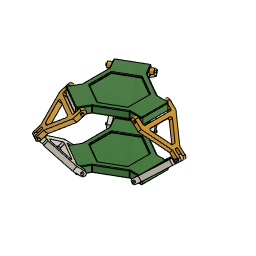
Triangular Podium v1 (Autodesk Fusion 360 design; units mm, degrees)
Autodesk Fusion 360 part; units mm, degrees
sketch "Sketch1" plane through (0, 0, 0) normal (0, 0, 1) x (1, 0, 0)
  line L0 (100, 57.735) -> (0, 115.4701)
  line L1 (0, 115.4701) -> (-100, 57.735)
  line L2 (-100, 57.735) -> (-100, -57.735)
  line L3 (-100, -57.735) -> (0, -115.4701)
  line L4 (0, -115.4701) -> (100, -57.735)
  line L5 (100, -57.735) -> (100, 57.735)
  line L6 (80, 46.188) -> (0, 92.376)
  line L7 (0, 92.376) -> (-80, 46.188)
  line L8 (-80, 46.188) -> (-80, -46.188)
  line L9 (-80, -46.188) -> (0, -92.376)
  line L10 (0, -92.376) -> (80, -46.188)
  line L11 (80, -46.188) -> (80, 46.188)
  dimension "d1" = 100
  dimension "d2" = 80
  measures "d1" distance of origin L5
  measures "d2" distance of origin L11
extrude "Extrude1" add sketch "Sketch1" along normal mid plane 20 contours L6 L7 L8 L9 L10 L11 makes body 1
extrude "Extrude2" add sketch "Sketch1" along normal mid plane 30 bodies 1
extrude "Extrude3" add 1 faces at (100, -19.245, -5) along direction (1, 0, 0) blind 50 on bodies 1 bodies 1
hole "Hole1" at (135, -57.735, 0) direction (0, 1, 0) diameter 10 end through all bodies 1
pattern_circular "C-Pattern1" count 3 over 360 about axis through (0, 0, 1.75) along (0, 0, 1) of "Extrude3", "Hole1"
fillet "Fillet1" radius 5 12 edges at (-25, -158.7713, 0) (-125, -101.0363, 0) (-100, -57.735, 0) (-100, 57.735, 0) (-125, 101.0363, 0) (-25, 158.7713, 0) (0, 115.4701, 0) (100, -57.735, 0) (0, -115.4701, 0) (150, -57.735, 0) (150, 57.735, 0) (100, 57.735, 0) on bodies 1
fillet "Fillet2" radius 2.5 2 faces at (-74.0032, -93.0206, 15) (-74.0032, -93.0206, -15) on bodies 1
cylinder "CylinderPrimitive1" add diameter 10 height -115.47 placed x (1, 0, 0) y (0, 0, 1) z (0, -1, 0) at (135, -57.735, 0) separate body makes body 2
move_face "OffsetFaces1" offset 20 1 faces at (136.3101, -57.735, -1.9935) on bodies 2
move_face "OffsetFaces2" offset 20 1 faces at (136.3101, 57.735, -1.9935) on bodies 2
pattern_circular "C-Pattern2" count 3 over 360 about axis through (0, 0, 1.75) along (0, 0, 1) of bodies 2 makes body 3 at (-45.856, 131.2484, 4.7396) makes body 4 at (-44.3828, -128.6965, 4.8131)
copy_body "Body->Comp1" bodies 1 removing the originals makes body 5 in component "Component"
copy_body "CutPasteBodies1" bodies 2 3 4 removing the originals makes body 6 makes body 7 makes body 8 in component "Component"
sketch "Sketch3" plane through (150, 0, 0) normal (1, 0, 0) x (0, 1, 0)
  line L0 (-52.735, -12.5) -> (52.735, -12.5)
  line L1 (52.735, -12.5) -> (52.735, 12.5)
  line L2 (52.735, 12.5) -> (-52.735, 12.5)
  line L3 (-52.735, 12.5) -> (-52.735, -12.5)
  line L4 (-77.735, 5) -> (-77.735, -5)
  line L5 (-57.735, 12.5) -> (-57.735, -12.5)
  line L6 (-52.735, -15) -> (52.735, -15)
  line L7 (57.735, -12.5) -> (57.735, 12.5)
  line L8 (77.735, -5) -> (77.735, 5)
  line L9 (-57.735, -15) -> (-72.735, -15)
  line L10 (-72.735, -15) -> (-72.735, 30)
  line L11 (-57.735, 20) -> (-57.735, -15)
  line L12 (-52.735, 25) -> (0, 25)
  line L13 (0, 25) -> (0, 100) construction
  line L14 (0, 130) -> (-15, 130)
  line L15 (-15, 130) -> (-72.735, 30)
  line L16 (0, 130) -> (15, 130)
  line L17 (15, 130) -> (72.735, 30)
  line L18 (72.735, -15) -> (72.735, 30)
  line L19 (57.735, -15) -> (72.735, -15)
  line L20 (57.735, 20) -> (57.735, -15)
  line L21 (52.735, 25) -> (0, 25)
  line L22 (40.9808, 40) -> (0, 40)
  line L23 (-40.9808, 40) -> (0, 40)
  line L24 (-6.3397, 115) -> (-45.3109, 47.5)
  line L25 (0, 115) -> (-6.3397, 115)
  line L26 (0, 115) -> (6.3397, 115)
  line L27 (6.3397, 115) -> (45.3109, 47.5)
  arc A0 (-45.3109, 47.5) -> (-40.9808, 40) centre (-40.9808, 45) ccw
  arc A1 (40.9808, 40) -> (45.3109, 47.5) centre (40.9808, 45) ccw
  arc A2 (-52.735, 25) -> (-57.735, 20) centre (-52.735, 20) ccw
  arc A3 (57.735, 20) -> (52.735, 25) centre (52.735, 20) ccw
  point P0 (-57.735, 25)
  dimension "d25" = 15
  dimension "d26" = 40
  dimension "d27" = 45
  dimension "d28" = 15
  dimension "d29" = 60
  dimension "d31" = 5
  constraint horizontal L9
  constraint vertical L10
  constraint vertical L11
  constraint vertical L5.end L9.start
  constraint horizontal L6.start L9.start
  constraint perpendicular L11 L12
  constraint perpendicular L0 L13
  constraint horizontal L14
  constraint vertical origin L14.start
  constraint symmetric L9.start L13 L19.start
  constraint symmetric L9.end L13 L18.start
  constraint symmetric L10.end L13 L17.end
  constraint symmetric L12.end L13 L21.end
  constraint symmetric L13 L14.start L16.start
  constraint symmetric L13 L14.end L16.end
  constraint tangent L23 A0
  constraint tangent L24 A0
  constraint tangent L22 A1
  constraint tangent L27 A1
  constraint equal A0 A1
  constraint coincident P0 L11
  constraint coincident P0 L12
  constraint tangent L11 A2
  constraint tangent L12 A2
  constraint equal A0 A2
  constraint tangent L20 A3
  constraint tangent L21 A3
  constraint equal A0 A3
  measures "d25" distance of L9.start L9.end
  measures "d26" distance of L9.start P0
  measures "d27" distance of L9.end L10.end
  measures "d28" distance of L14.start L14.end
  measures "d29" angle of L12 L15
  measures "d31" radius of A0
extrude "Extrude1'" add sketch "Sketch3" along normal blind 20 separate body contours L5 L7 L9 L10 L11 L12 L14 L15 L16 L17 L18 L19 L20 L21 A2 A3 makes body 9 in component "Component'"
hole "Hole1'" at (160, -72.735, 0) direction (0, 1, 0) diameter 10 end through all bodies 9 in component "Component'"
fillet "Fillet1'" radius 10 4 edges at (170, -65.235, -15) (150, -65.235, -15) (170, 65.235, -15) (150, 65.235, -15) on bodies 9 in component "Component'"
extrude "Extrude1''" add sketch "Sketch3" along normal blind 20 separate body contours L5 L7 L9 L10 L11 L12 L14 L15 L16 L17 L18 L19 L20 L21 A2 A3 makes body 10 in component "Component''"
hole "Hole1''" at (160, -72.735, 0) direction (0, 1, 0) diameter 10 end through all bodies 10 in component "Component''"
fillet "Fillet1''" radius 10 4 edges at (170, -65.235, -15) (150, -65.235, -15) (170, 65.235, -15) (150, 65.235, -15) on bodies 10 in component "Component''"
sketch "Sketch4" plane through (0, 0, 0) normal (0, 1, 0) x (1, 0, 0)
  line L0 (150, -130) -> (170, -130)
  line L1 (225, -130) -> (245, -130)
  line L2 (150, -130) -> (170, -130)
  line L3 (170, -130) -> (170, -160)
  line L4 (150, -160) -> (150, -130)
  line L5 (225, -130) -> (245, -130)
  line L6 (245, -130) -> (245, -160)
  line L7 (225, -160) -> (225, -130)
  circle A0 centre (160, -160) radius 5
  arc A1 (150, -160) -> (170, -160) centre (160, -160) ccw
  circle A2 centre (235, -160) radius 5
  arc A3 (225, -160) -> (245, -160) centre (235, -160) ccw
  dimension "d40" = 20
  dimension "d41" = 30
  dimension "d42" = 20
  dimension "d43" = 30
  dimension "d44" = 20
  dimension "d45" = 10
  dimension "d46" = 20
  dimension "d47" = 10
  constraint horizontal L2
  constraint vertical L3
  constraint vertical L4
  constraint coincident L0.start L2.start
  constraint horizontal L5
  constraint vertical L6
  constraint vertical L7
  constraint coincident L1.start L5.start
  constraint concentric A0 A1
  constraint concentric A2 A3
  measures "d40" distance of L0.start L0.end
  measures "d41" distance of L0.start L4.start
  measures "d42" distance of L1.start L1.end
  measures "d43" distance of L1.start L7.start
  measures "d44" diameter of A1
  measures "d45" diameter of A0
  measures "d46" diameter of A3
  measures "d47" diameter of A2
extrude "Extrude2'" add sketch "Sketch4" along normal mid plane 10 contours L0 L2 L3 L4 A1 bodies 9 in component "Component'"
extrude "Extrude2''" add sketch "Sketch4" along normal blind 10 from surface at 5 contours L1 L5 L6 L7 A3 sketch seen with x (1, 0, 0) y (0, 1, 0) z (0, 0, 1) at (-75, 0, 0) bodies 10 in component "Component''"
mirror "Mirror1" about plane through (-75, 0, 0) normal (0, 1, 0) of "Extrude2''" in component "Component''"
cylinder "CylinderPrimitive1'" add diameter 10 height 40 placed x (1, 0, 0) y (0, 0, 1) z (0, -1, 0) at (160, -5, 160) separate body makes body 11 in component "Component'''"
move_body "Move1" bodies 11 to x (1, 0, 0) y (0, 1, 0) z (0, 0, 1) at (0, 25, 0) in component "Component'''"
component_pattern "component pattern"
component "Component" placed x (1, 0, 0) y (0, 1, 0) z (0, 0, 1) at (0, 0, 0)
component "Component'" placed x (1, 0, 0) y (0, 1, 0) z (0, 0, 1) at (-25, 0, 0)
component "Component''" placed x (-1, 0, 0) y (0, 1, 0) z (0, 0, -1) at (295, 0, 320)
component "Component'''" placed x (-0.99999, 0, -0.004441) y (0, 1, 0) z (0.004441, 0, -0.99999) at (294.2879, 0, 320.7089)
component "Component'" placed x (-0.5, 0.866025, 0) y (-0.866025, -0.5, 0) z (0, 0, 1) at (12.5, -21.6506, 0)
component "Component''" placed x (0.5, -0.866025, 0) y (-0.866025, -0.5, 0) z (0, 0, -1) at (-147.5, 255.4775, 320)
component "Component'''" placed x (0.5, -0.866025, 0) y (-0.866025, -0.5, 0) z (0, 0, -1) at (-147.5, 255.4775, 320)
component "Component'" placed x (-0.5, -0.866025, 0) y (0.866025, -0.5, 0) z (0, 0, 1) at (12.5, 21.6506, 0)
component "Component''" placed x (0.5, 0.866025, 0) y (0.866025, -0.5, 0) z (0, 0, -1) at (-147.5, -255.4775, 320)
component "Component'''" placed x (0.5, 0.866025, 0) y (0.866025, -0.5, 0) z (0, 0, -1) at (-147.5, -255.4775, 320)
component "Component" placed x (1, 0, 0) y (0, 1, 0) z (0, 0, 1) at (0, 0, 320)
